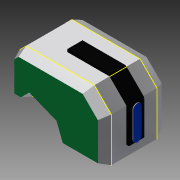
# Autodesk Inventor part: Head
Saved by Autodesk Inventor 2014 (Build 180170000, 170)
## iProperties
Created: 2016-12-21
Part Number: Head
Material: Generic
Document SubType Name: Modeling
Designer: lloi
Density: 1 g/cm^3
Appearance: Default
Author: lloi
Autodesk Inventor part; units mm, degrees
ref_plane "YZ Plane" through (0, 0, 0) normal (1, 0, 0) x (0, 1, 0)
sketch "Sketch1" plane through (0, 0, 0) normal (0, 0, 1) x (1, 0, 0)
  line L0 (-118.4529, 91.44) -> (86.7029, 91.44)
  line L1 (137.5029, 40.64) -> (137.5029, -91.44)
  line L2 (137.5029, -91.44) -> (10.5029, -91.44)
  line L3 (-137.5029, -30.1879) -> (-137.5029, 72.39)
  line L4 (-137.5029, 72.39) -> (-137.5029, -30.1879)
  line L5 (86.7029, 91.44) -> (137.5029, 40.64)
  line L6 (-118.4529, 91.44) -> (-137.5029, 72.39)
  line L7 (137.5029, -91.44) -> (10.5029, -91.44)
  line L8 (10.5029, -91.44) -> (-8.146196, -40.20203)
  line L9 (10.5029, -91.44) -> (65.029209, -91.44) construction
  line L10 (-8.146196, -40.20203) -> (-79.70483, -12.227388)
  line L11 (-79.70483, -12.227388) -> (-97.665343, -30.1879)
  line L12 (-97.665343, -30.1879) -> (-137.5029, -30.1879)
  constraints: 26 end point, 4 parallel, 2 horizontal, 2 perpendicular, 1 equal length
extrude "Extrusion1" add sketch "Sketch1" along normal mid plane 137.16
sketch "Sketch2" plane through (0, 0, -68.58) normal (0, 0, -1) x (-1, 0, 0)
  line L0 (-137.5029, 40.64) -> (-137.5029, -91.44)
  line L1 (-137.5029, -91.44) -> (-10.5029, -91.44)
  line L2 (-10.5029, -91.44) -> (8.146196, -40.20203)
  line L3 (8.146196, -40.20203) -> (79.70483, -12.227388)
  line L4 (79.70483, -12.227388) -> (97.665343, -30.1879)
  line L5 (97.665343, -30.1879) -> (137.5029, -30.1879)
  line L6 (137.5029, -30.1879) -> (137.5029, 72.39)
  line L7 (137.5029, 72.39) -> (118.4529, 91.44)
  line L8 (118.4529, 91.44) -> (-86.7029, 91.44)
  line L9 (-86.7029, 91.44) -> (-137.5029, 40.64)
  point P0 (0, 0)
sketch "Sketch3" plane through (0, 0, 68.58) normal (0, 0, 1) x (1, 0, 0)
  line L0 (137.5029, -91.44) -> (137.5029, 40.64)
  line L1 (137.5029, 40.64) -> (86.7029, 91.44)
  line L2 (86.7029, 91.44) -> (-118.4529, 91.44)
  line L3 (-118.4529, 91.44) -> (-137.5029, 72.39)
  line L4 (-137.5029, 72.39) -> (-137.5029, -30.1879)
  line L5 (-137.5029, -30.1879) -> (-97.665343, -30.1879)
  line L6 (-97.665343, -30.1879) -> (-79.70483, -12.227388)
  line L7 (-79.70483, -12.227388) -> (-8.146196, -40.20203)
  line L8 (-8.146196, -40.20203) -> (10.5029, -91.44)
  line L9 (10.5029, -91.44) -> (137.5029, -91.44)
  point P0 (0, 0)
ref_plane "Work Plane1" through (0, 0, 96.012) normal (0, 0, 1) x (1, 0, 0)
ref_plane "Work Plane2" through (0, 0, -96.012) normal (0, 0, -1) x (-1, 0, 0)
sketch "Sketch4" plane through (0, 0, 96.012) normal (0, 0, 1) x (1, 0, 0)
  line L0 (-126.464731, 65.844437) -> (-126.464731, -22.902911)
  line L1 (-126.464731, -22.902911) -> (-106.411156, -22.902911)
  line L2 (-106.411156, -22.902911) -> (-89.052252, -5.544007)
  line L3 (-106.411156, -22.902911) -> (-81.511939, 1.996306)
  line L4 (-81.511939, 1.996306) -> (0.53602, -30.665165)
  line L5 (0.53602, -30.665165) -> (19.270518, -79.10194)
  line L6 (19.270518, -79.10194) -> (124.736838, -79.10194)
  line L7 (124.736838, -79.10194) -> (124.736838, 33.064062)
  line L8 (124.736838, 33.064062) -> (79.026361, 78.774539)
  line L9 (79.026361, 78.774539) -> (-113.534629, 78.774539)
  line L10 (-113.534629, 78.774539) -> (-126.464731, 65.844437)
  point P0 (0, 0)
  constraints: 22 end point, 4 perpendicular, 2 parallel, 1 collinear, 1 vertical
sketch "Sketch4 outline for Loft1" plane through (0, 0, 96.012) normal (0, 0, 1) x (1, 0, 0)
  line L0 (-113.534629, 78.774539) -> (-126.464731, 65.844437)
  line L1 (79.026361, 78.774539) -> (-113.534629, 78.774539)
  line L2 (124.736838, 33.064062) -> (79.026361, 78.774539)
  line L3 (124.736838, -79.10194) -> (124.736838, 33.064062)
  line L4 (19.270518, -79.10194) -> (124.736838, -79.10194)
  line L5 (0.53602, -30.665165) -> (19.270518, -79.10194)
  line L6 (-81.511939, 1.996306) -> (0.53602, -30.665165)
  line L7 (-106.411156, -22.902911) -> (-81.511939, 1.996306)
  line L8 (-126.464731, -22.902911) -> (-106.411156, -22.902911)
  line L9 (-126.464731, 65.844437) -> (-126.464731, -22.902911)
loft "Loft1" add profiles "Sketch4 outline for Loft1" section 2 edges at (137.5029, -25.4, 68.58) (112.1029, 66.04, 68.58) (-15.875, 91.44, 68.58) (-127.9779, 81.915, 68.58) (-137.5029, 21.10105, 68.58) (-117.584121, -30.1879, 68.58) (-88.685086, -21.207644, 68.58) (-43.925513, -26.214709, 68.58) (1.178352, -65.821015, 68.58) (74.0029, -91.44, 68.58)
sketch "Sketch5" plane through (-113.534629, 78.774539, 96.012) normal (0, 0, 1) x (1, 0, 0)
  line L0 (-12.930103, -12.930103) -> (-12.930103, -101.67745)
  line L1 (-12.930103, -101.67745) -> (7.123473, -101.67745)
  line L2 (7.123473, -101.67745) -> (32.02269, -76.778233)
  line L3 (32.02269, -76.778233) -> (114.070648, -109.439704)
  line L4 (114.070648, -109.439704) -> (132.805147, -157.876479)
  line L5 (132.805147, -157.876479) -> (238.271467, -157.876479)
  line L6 (238.271467, -157.876479) -> (238.271467, -45.710478)
  line L7 (238.271467, -45.710478) -> (192.560989, 0)
  line L8 (192.560989, 0) -> (0, 0)
  line L9 (0, 0) -> (-12.930103, -12.930103)
  point P0 (113.534629, -78.774539)
extrude "Extrusion2" add sketch "Sketch5" against normal blind 192.024
loft "Loft2" add section 1 edges at (-126.464731, 21.470763, -96.012) (-119.99968, 72.309488, -96.012) (-17.254134, 78.774539, -96.012) (101.881599, 55.9193, -96.012) (124.736838, -23.018939, -96.012) (72.003678, -79.10194, -96.012) (9.903269, -54.883552, -96.012) (-40.487959, -14.33443, -96.012) (-93.961547, -10.453303, -96.012) (-116.437944, -22.902911, -96.012) section 2 edges at (137.5029, -25.4, -68.58) (74.0029, -91.44, -68.58) (1.178352, -65.821015, -68.58) (-43.925513, -26.214709, -68.58) (-88.685086, -21.207644, -68.58) (-117.584121, -30.1879, -68.58) (-137.5029, 21.10105, -68.58) (-127.9779, 81.915, -68.58) (-15.875, 91.44, -68.58) (112.1029, 66.04, -68.58)
sketch "Sketch6" plane through (86.7029, 91.44, -68.58) normal (0.7071068, 0.7071068, 0) x (-0.7071068, 0.7071068, 0)
  line L0 (0, 0) -> (0, 137.16)
  line L1 (-71.842049, 0) -> (-71.842049, 137.16)
  line L2 (0, 137.16) -> (0, 91.44)
  line L3 (-71.842049, 0) -> (-71.842049, 45.72)
  line L4 (-71.842049, 45.72) -> (0, 45.72)
  line L5 (0, 45.72) -> (0, 91.44)
  line L6 (0, 91.44) -> (-71.842049, 91.44)
  line L7 (-71.842049, 91.44) -> (-71.842049, 45.72)
  point P0 (-3.349636, 68.58)
  dimension "d44" = 45.72
  dimension "d45" = 45.72
  constraints: 12 end point, 2 parallel, 2 point on line, 1 horizontal, 1 perpendicular
  measures "d44" distance of L0.end L2.end
  measures "d45" distance of L1.start L3.end
extrude "Extrusion3" add sketch "Sketch6" along normal blind 7.62
sketch "Sketch7" plane through (-118.4529, 91.44, 68.58) normal (0, 1, 0) x (1, 0, 0)
  line L0 (0, 137.16) -> (0, 0) projected
  line L1 (0, 137.16) -> (0, 91.44)
  line L2 (205.1558, 0) -> (205.1558, 45.72)
  line L3 (205.1558, 45.72) -> (78.1558, 45.72)
  line L4 (78.1558, 45.72) -> (78.1558, 91.44)
  line L5 (78.1558, 91.44) -> (205.1558, 91.44)
  line L6 (205.1558, 91.44) -> (205.1558, 45.72)
  point P0 (118.4529, 68.58)
  dimension "d48" = 45.72
  dimension "d49" = 127
  constraints: 12 end point, 3 parallel, 1 horizontal, 1 perpendicular, 1 point on line
  measures "d48" distance of L0.start L1.end
  measures "d49" distance of L4.end L5.end
extrude "Extrusion4" add sketch "Sketch7" along normal blind 7.62
sketch "Sketch8" plane through (137.5029, -91.44, 68.58) normal (1, 0, 0) x (0, 0, -1)
  line L0 (45.72, 132.08) -> (91.44, 132.08)
  line L1 (91.44, 132.08) -> (91.44, 30.48)
  line L2 (91.44, 30.48) -> (45.72, 30.48)
  line L3 (45.72, 30.48) -> (45.72, 132.08)
  point P0 (68.58, 91.44)
  dimension "d52" = 101.6
  constraints: 8 end point, 2 parallel, 1 horizontal, 1 perpendicular
  measures "d52" distance of L0.end L1.end
extrude "Extrusion5" add sketch "Sketch8" along normal blind 7.62
sketch "Sketch9" plane through (92.091054, 96.828154, -22.86) normal (-0.7071068, 0.7071068, 0) x (-0.7071068, -0.7071068, 0)
  line L0 (7.62, 0) -> (7.62, 45.72) projected
  line L1 (7.62, 45.72) -> (0, 45.72) projected
  line L2 (0, 0) -> (0, 45.72) projected
  line L3 (7.62, 0) -> (0, 0) projected
  point P0 (133.586053, 22.86)
sketch "Sketch10" plane through (142.891054, 46.028154, 22.86) normal (0, 0, 1) x (0.7071068, 0.7071068, 0)
  line L0 (-7.62, 0) -> (-7.62, 71.842049)
  line L1 (-7.62, 0) -> (0, 0)
  line L2 (0, 71.842049) -> (0, 0)
  line L3 (-7.62, 71.842049) -> (0, 71.842049)
  line L4 (-7.62, 71.842049) -> (-2.257751, 77.255983)
  line L5 (-7.62, 0) -> (-2.231846, -5.388154)
  line L6 (-7.62, 0) -> (0, 0) construction
  line L7 (-2.231846, -5.388154) -> (0, 0)
  line L8 (-2.257751, 77.255983) -> (0, 71.842049)
  line L9 (0, 71.842049) -> (0, 0)
  point P0 (-133.586053, 68.492413)
  dimension "d55" = 7.62
  dimension "d56" = 7.62
  dimension "d57" = 45
  constraints: 12 end point, 1 equal length, 1 horizontal
  measures "d55" distance of L0.end L4.end
  measures "d56" distance of L0.start L5.end
  measures "d57" angle of L5 L6
extrude "Extrusion6" add sketch "Sketch10" against normal blind 45.72
sketch "Sketch11" plane through (145.1229, -91.44, 68.58) normal (1, 0, 0) x (0, 0, -1)
  line L0 (45.72, 30.48) -> (91.44, 30.48) projected
  line L1 (91.44, 132.08) -> (45.72, 132.08) projected
  line L2 (68.58, 132.08) -> (68.58, 30.48) construction
  line L3 (55.88, 119.38) -> (55.88, 43.18)
  line L4 (81.28, 43.18) -> (81.28, 119.38)
  arc A0 (81.28, 119.38) -> (55.88, 119.38) centre (68.58, 119.38) ccw
  arc A1 (55.88, 43.18) -> (81.28, 43.18) centre (68.58, 43.18) ccw
  point P0 (68.58, 91.44)
  point P1 (68.58, 81.28)
  dimension "d60" = 25.4
  constraints: 8 end point, 6 point on circle, 4 tangent, 3 midpoint, 2 centre point, 2 point on line, 1 parallel
  measures "d60" diameter of A1
extrude "Extrusion7" add sketch "Sketch11" along normal blind 2.54
body "Solid1"
